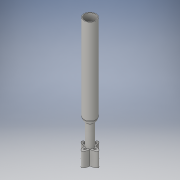
# Autodesk Inventor part: BB-8_headslider_stilt
Saved by Autodesk Inventor 2016 (Build 200138000, 138)
## iProperties
Created: 2018-07-16
Part Number: BB-8_headslider_stilt
Material: Generic
Document SubType Name: Modeling
Designer: Karcsi
Density: 1 g/cm^3
Appearance: Default
Author: Karcsi
Autodesk Inventor part; units mm, degrees
ref_plane "YZ Plane" through (0, 0, 0) normal (1, 0, 0) x (0, 1, 0)
ref_plane "XZ Plane" through (0, 0, 0) normal (0, 1, 0) x (-1, 0, 0)
ref_plane "XY Plane" through (0, 0, 0) normal (0, 0, 1) x (1, 0, 0)
sketch "Sketch1" plane through (0, 0, 0) normal (0, 1, 0) x (-1, 0, 0)
  ellipse E0 centre (0, 0) end of major axis (0, 11.8) minor radius 4.3
  ellipse E1 centre (0, 0) end of major axis (11.8, 0) minor radius 4.3
  dimension "d0" = 11.8
  dimension "d1" = 4.3
  dimension "d2" = 11.8
  dimension "d3" = 4.3
  constraints: 2 coincident, 4 other
sketch "Sketch2" plane through (0, 0, 0) normal (0, 1, 0) x (-1, 0, 0)
  circle A0 centre (7, 0) radius 1.5
  circle A1 centre (0, -7) radius 1.5
  circle A2 centre (-7, 0) radius 1.5
  circle A3 centre (0, 7) radius 1.5
  point P0 (0, 0)
  dimension "d4" = 3
  dimension "d5" = 3
  dimension "d6" = 3
  dimension "d7" = 3
  dimension "d8" = 7
  dimension "d9" = 7
  dimension "d10" = 7
  dimension "d11" = 7
  constraints: 4 centre point
  measures "d4" diameter of A0
  measures "d5" diameter of A1
  measures "d6" diameter of A2
  measures "d7" diameter of A3
  measures "d8" distance of point (0, 0) A0.centre
  measures "d9" distance of point (0, 0) A1.centre
  measures "d10" distance of point (0, 0) A2.centre
  measures "d11" distance of point (0, 0) A3.centre
extrude "Extrusion1" add sketch "Sketch1" along normal blind 20
hole "Hole1" at (7, 0, 0) at (0, 0, 7) at (0, 0, -7) at (-7, 0, 0) direction (0, 1, 0) diameter 3 depth 20 tip angle 118
sketch "Sketch5" plane through (0, 20, 0) normal (0, 1, 0) x (1, 0, 0)
  circle A0 centre (0, 0) radius 5
  circle A1 centre (0, 0) radius 3
  dimension "d25" = 10
  dimension "d26" = 6
  constraints: 2 centre point, 2 coincident
  measures "d25" diameter of A0
  measures "d26" diameter of A1
extrude "Extrusion3" add sketch "Sketch5" along normal blind 30
sketch "Sketch6" plane through (0, 50, 0) normal (0, 1, 0) x (1, 0, 0)
  point P0 (0, 0)
sketch "Sketch7" plane through (0, 50, 0) normal (0, 1, 0) x (1, 0, 0)
  circle A0 centre (0, 0) radius 8
  dimension "d29" = 16
  constraints: 1 centre point, 1 coincident
  measures "d29" diameter of A0
extrude "Extrusion4" add sketch "Sketch7" along normal blind 5
fillet "Fillet1" radius 6.7625 1 edges at (-8, 50, 0)
sketch "Sketch8" plane through (0, 55, 0) normal (0, 1, 0) x (1, 0, 0)
  circle A0 centre (0, 0) radius 8.5
  circle A1 centre (0, 0) radius 7.5
  dimension "d33" = 17
  dimension "d34" = 15
  constraints: 2 centre point, 2 coincident
  measures "d33" diameter of A0
  measures "d34" diameter of A1
sketch "Sketch9" plane through (0, 55, 0) normal (0, 1, 0) x (1, 0, 0)
  circle A0 centre (0, 0) radius 5.75
  circle A1 centre (0, 0) radius 4.75
  dimension "d35" = 11.5
  dimension "d36" = 9.5
  constraints: 2 centre point, 2 coincident
  measures "d35" diameter of A0
  measures "d36" diameter of A1
extrude "Extrusion5" add sketch "Sketch8" along normal blind 120
extrude "Extrusion6" add sketch "Sketch9" along normal blind 20
sketch "Sketch10" plane through (0, 75, 0) normal (0, 1, 0) x (1, 0, 0)
  point P0 (0, 0)
sketch "Sketch11" plane through (0, 75, 0) normal (0, 1, 0) x (1, 0, 0)
  point P0 (0, 0)
fillet "Fillet4" radius 2 1 edges at (-8.5, 55, 0)
body "Solid1"
